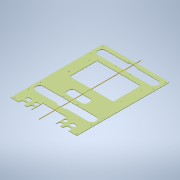
# Autodesk Inventor part: out_front
Saved by Autodesk Inventor 2020.2 (Build 242310000, 310)
## iProperties
Created: 2017-08-14
Part Number: out_front
Material: 一般
Document SubType Name: Modeling
Designer: gisen
Density: 1 g/cm^3
Appearance: クロム酸亜鉛 2
Author: gisen
Autodesk Inventor part; units mm, degrees
note: some values were not read from the file. Chosen so that the rebuilt part matches the saved one: offset side.
ref_plane "YZ Plane" through (0, 0, 0) normal (1, 0, 0) x (0, 1, 0)
ref_plane "XZ Plane" through (0, 0, 0) normal (0, 1, 0) x (-1, 0, 0)
ref_plane "XY Plane" through (0, 0, 0) normal (0, 0, 1) x (1, 0, 0)
sketch "スケッチ1" plane through (0, 0, 0) normal (0, 0, 1) x (1, 0, 0)
  line L0 (-165, 165) -> (165, 165)
  line L1 (165, 165) -> (165, -165)
  line L2 (165, -165) -> (-165, -165)
  line L3 (-165, -165) -> (-165, 165)
  line L4 (-165, 165) -> (165, -165) construction
  line L5 (165, 165) -> (-165, -165) construction
  circle A0 centre (-155, 155) radius 1.6
  circle A1 centre (-155, -155) radius 1.6
  circle A2 centre (155, -155) radius 1.6
  circle A3 centre (155, 155) radius 1.6
  point P0 (0, 0)
  dimension "d0" = 330
  dimension "d1" = 330
  dimension "d2" = 3.2
  dimension "d3" = 3.2
  dimension "d4" = 3.2
  dimension "d5" = 3.2
  dimension "d6" = 10
  dimension "d7" = 10
  dimension "d8" = 10
  dimension "d9" = 10
  constraints: 12 end point, 4 centre point, 4 point on line, 2 midpoint, 2 parallel, 1 horizontal, 1 perpendicular
  measures "d0" distance of L1.end L2.end
  measures "d1" distance of L0.end L1.end
  measures "d2" diameter of A0
  measures "d3" diameter of A1
  measures "d4" diameter of A2
  measures "d5" diameter of A3
  measures "d6" distance from line of A0.centre L0
  measures "d7" distance from line of L2 A1.centre
  measures "d8" distance from line of L2 A2.centre
  measures "d9" distance from line of L0 A3.centre
extrude "押し出し1" add sketch "スケッチ1" along normal blind 2
sketch "スケッチ2" plane through (0, 0, 2) normal (0, 0, 1) x (1, 0, 0)
  circle A0 centre (155, 155) radius 1.6 construction
  circle A1 centre (155, -155) radius 1.6 construction
  circle A2 centre (-155, -155) radius 1.6 construction
  circle A3 centre (-155, 155) radius 1.6 construction
  line L0 (165, 165) -> (-165, 165) construction
  line L1 (-165, 165) -> (-165, -165) construction
  line L2 (-165, -165) -> (165, -165) construction
  line L3 (165, -165) -> (165, 165) construction
  line L4 (165, 165) -> (-165, 165) construction
  line L5 (0, 165) -> (0, -165) construction
  line L6 (-108.5, 102) -> (108.5, 102)
  line L7 (108.5, 102) -> (108.5, -35)
  line L8 (108.5, -35) -> (-108.5, -35)
  line L9 (-108.5, -35) -> (-108.5, 102)
  line L10 (-108.5, 102) -> (108.5, -35) construction
  line L11 (108.5, 102) -> (-108.5, -35) construction
  line L12 (-125, -55) -> (125, -55)
  line L13 (125, -55) -> (125, -119.5)
  line L14 (125, -119.5) -> (-125, -119.5)
  line L15 (-125, -119.5) -> (-125, -55)
  line L16 (-125, -55) -> (125, -119.5) construction
  line L17 (125, -55) -> (-125, -119.5) construction
  point P0 (0, 0)
  point P1 (0, 33.5)
  point P2 (0, -87.25)
  dimension "d12" = 63
  dimension "d13" = 217
  dimension "d14" = 137
  dimension "d15" = 20
  dimension "d16" = 64.5
  dimension "d17" = 250
  constraints: 26 end point, 6 midpoint, 4 parallel, 2 horizontal, 2 perpendicular, 2 point on line
  measures "d12" distance between parallel lines of L6 L0
  measures "d13" distance of L6.start L6.end
  measures "d14" distance of L6.end L7.end
  measures "d15" distance between parallel lines of L12 L8
  measures "d16" distance of L12.end L13.end
  measures "d17" distance of L13.end L14.end
extrude "押し出し2" cut sketch "スケッチ2" against normal through all
sketch "スケッチ3" plane through (0, 0, 0) normal (0, 0, -1) x (-1, 0, 0)
  line L0 (108.5, 102) -> (108.5, -35) construction
  line L1 (-108.5, -35) -> (-108.5, 102) construction
  line L2 (108.5, -35) -> (108.5, 102) construction
  line L3 (108.5, -35) -> (-108.5, 102) construction
  line L4 (-108.5, -35) -> (108.5, 102) construction
  line L5 (122.5, 105.5) -> (-122.5, 105.5) construction
  line L6 (-122.5, 105.5) -> (-122.5, -38.5) construction
  line L7 (-122.5, -38.5) -> (122.5, -38.5) construction
  line L8 (122.5, -38.5) -> (122.5, 105.5) construction
  line L9 (122.5, 105.5) -> (-122.5, -38.5) construction
  line L10 (-122.5, 105.5) -> (122.5, -38.5) construction
  line L11 (165, 165) -> (-165, 165) construction
  circle A0 centre (129.75, -16.5) radius 2
  line L12 (0, -38.5) -> (0, 165) construction
  line L13 (-122.5, -38.5) -> (-122.5, 105.5) construction
  circle A1 centre (-129.75, -16.5) radius 2
  circle A2 centre (129.75, 83.5) radius 2
  circle A3 centre (-129.75, 83.5) radius 2
  circle A4 centre (129.75, 93) radius 1.5
  circle A5 centre (129.75, 74) radius 1.5
  circle A6 centre (129.75, -7) radius 1.5
  circle A7 centre (129.75, -26) radius 1.5
  circle A8 centre (-129.75, -26) radius 1.5
  circle A9 centre (-129.75, -7) radius 1.5
  circle A10 centre (-129.75, 74) radius 1.5
  circle A11 centre (-129.75, 93) radius 1.5
  point P0 (0, 0)
  point P1 (0, 33.5)
  dimension "d20" = 245
  dimension "d21" = 144
  dimension "d26" = 22
  dimension "d27" = 7.25
  dimension "d30" = 7.25
  dimension "d33" = 7.25
  dimension "d71" = 4
  dimension "d72" = 22
  dimension "d73" = 22
  dimension "d74" = 4
  dimension "d75" = 4
  dimension "d76" = 3
  dimension "d77" = 3
  dimension "d78" = 3
  dimension "d79" = 3
  dimension "d80" = 3
  dimension "d81" = 3
  dimension "d82" = 3
  dimension "d83" = 3
  dimension "d84" = 9.5
  dimension "d86" = 9.5
  dimension "d87" = 9.5
  dimension "d88" = 9.5
  dimension "d89" = 9.5
  dimension "d90" = 9.5
  dimension "d91" = 9.5
  dimension "d92" = 9.5
  constraints: 20 end point, 12 centre point, 8 vertical alignment, 5 midpoint, 2 parallel, 1 horizontal, 1 perpendicular, 1 symmetric about line
  measures "d20" distance of L7.end L6.end
  measures "d21" distance of L5.end L6.end
  measures "d26" distance from line of A0.centre L7
  measures "d27" distance from line of L8 A0.centre
  measures "d30" distance from line of L8 A2.centre
  measures "d33" distance from line of L6 A3.centre
  measures "d71" diameter of A1
  measures "d72" distance from line of L5 A2.centre
  measures "d73" distance from line of L5 A3.centre
  measures "d74" diameter of A3
  measures "d75" diameter of A2
  measures "d76" diameter of A4
  measures "d77" diameter of A5
  measures "d78" diameter of A6
  measures "d79" diameter of A7
  measures "d80" diameter of A8
  measures "d81" diameter of A9
  measures "d82" diameter of A10
  measures "d83" diameter of A11
  measures "d84" distance of A3.centre A11.centre
  measures "d86" distance of A3.centre A10.centre
  measures "d87" distance of A1.centre A9.centre
  measures "d88" distance of A1.centre A8.centre
  measures "d89" distance of A0.centre A7.centre
  measures "d90" distance of A0.centre A6.centre
  measures "d91" distance of A2.centre A4.centre
  measures "d92" distance of A2.centre A5.centre
extrude "押し出し3" cut sketch "スケッチ3" against normal through all contours A0 | A1 | A2 | A3
sketch "スケッチ4" plane through (0, 0, 2) normal (0, 0, 1) x (1, 0, 0)
  line L0 (165, -165) -> (165, 165) projected
  line L1 (-165, -165) -> (165, -165)
  line L2 (165, -165) -> (165, -272)
  line L3 (165, -272) -> (-165, -272)
  line L4 (-165, -272) -> (-165, -165)
  circle A0 centre (-155, 155) radius 1.6 projected
  circle A1 centre (155, 155) radius 1.6 projected
  circle A2 centre (-155, -155) radius 1.6 projected
  circle A3 centre (155, -155) radius 1.6 projected
  circle A4 centre (-155, -262) radius 2.5
  circle A5 centre (155, -262) radius 2.5
  circle A6 centre (-155, 178) radius 2.5
  circle A7 centre (155, 178) radius 2.5
  line L5 (-165, 188) -> (165, 188)
  line L6 (165, 188) -> (165, 165)
  line L7 (165, 165) -> (-165, 165)
  line L8 (-165, 165) -> (-165, 188)
  point P0 (0, 0)
  dimension "d35" = 107
  dimension "d40" = 10
  dimension "d41" = 10
  dimension "d42" = 5
  dimension "d43" = 5
  dimension "d44" = 5
  dimension "d45" = 5
  dimension "d46" = 10
  dimension "d47" = 10
  dimension "d48" = 23
  dimension "d49" = 10
  dimension "d50" = 10
  dimension "d51" = 10
  dimension "d52" = 10
  constraints: 16 end point, 4 centre point, 4 parallel, 2 horizontal, 2 perpendicular, 2 point on line, 1 coincident
  measures "d35" distance of L1.end L2.end
  measures "d40" distance from line of L3 A4.centre
  measures "d41" distance from line of L4 A4.centre
  measures "d42" diameter of A6
  measures "d43" diameter of A7
  measures "d44" diameter of A5
  measures "d45" diameter of A4
  measures "d46" distance from line of L3 A5.centre
  measures "d47" distance from line of L2 A5.centre
  measures "d48" distance of L7.end L5.start
  measures "d49" distance from line of A6.centre L5
  measures "d50" distance from line of L8 A6.centre
  measures "d51" distance from line of L5 A7.centre
  measures "d52" distance from line of L6 A7.centre
extrude "押し出し4" add sketch "スケッチ4" against normal up to surface (2 mm away)
sketch "スケッチ8" plane through (0, 0, 0) normal (0, 0, -1) x (-1, 0, 0)
  circle A0 centre (-72.25, -236.56) radius 7.94 projected
  circle A1 centre (-72.25, -262.06) radius 7.94 projected
  circle A2 centre (72.25, -236.24) radius 7.44 projected
  circle A3 centre (72.25, -261.74) radius 7.44 projected
  line L0 (29, -272) -> (29, -227) projected
  line L1 (29, -227) -> (-31, -227) projected
  line L2 (-31, -227) -> (-31, -272) projected
  ellipse E0 centre (-109.425, -236.08) end of major axis (-121.4458, -236.08) minor radius 8.5 projected
  ellipse E1 centre (-109.425, -262.32) end of major axis (-121.4458, -262.32) minor radius 8.5 projected
  ellipse E2 centre (109.425, -236.08) end of major axis (121.4458, -236.08) minor radius 8.5 projected
  ellipse E3 centre (109.425, -262.32) end of major axis (121.4458, -262.32) minor radius 8.5 projected
  point P0 (0, 0)
  constraints: 4 other
extrude "押し出し8" cut sketch "スケッチ8" against normal blind 10
sketch "スケッチ9" plane through (0, 0, 0) normal (0, 0, -1) x (-1, 0, 0)
  line L0 (-31, -227) -> (-31, -272) projected
  line L1 (29, -227) -> (-31, -227) projected
  line L2 (29, -272) -> (29, -227) projected
  line L3 (-31, -272) -> (29, -272)
  line L4 (165, -272) -> (-165, -272) projected
  point P0 (0, 0)
  constraints: 2 end point, 1 collinear
extrude "押し出し9" cut sketch "スケッチ9" against normal blind 10
sketch "スケッチ13" plane through (0, 0, 2) normal (0, 0, 1) x (1, 0, 0)
  line L0 (-130, -162.3) -> (130, -162.3) construction
  line L1 (-130, -142.3) -> (130, -142.3)
  line L2 (130, -182.3) -> (-130, -182.3)
  arc A0 (-130, -142.3) -> (-130, -182.3) centre (-130, -162.3) ccw
  arc A1 (130, -182.3) -> (130, -142.3) centre (130, -162.3) ccw
  line L3 (-165, -272) -> (-29, -272) projected
  point P0 (0, 0)
  point P1 (0, -162.3)
  dimension "d116" = 40
  dimension "d117" = 0
  dimension "d118" = 260
  dimension "d119" = 129.7
  constraints: 8 end point, 4 point on circle, 4 tangent, 2 centre point, 1 horizontal, 1 midpoint, 1 parallel
  measures "d116" diameter of A0
  measures "d117" horizontal distance of point (0, 0) point (0, -162.3)
  measures "d118" distance of L0.end L0.start
  measures "d119" distance between parallel lines of L1 L3
extrude "押し出し13" cut sketch "スケッチ13" against normal through all
sketch "スケッチ14" plane through (0, 0, 2) normal (0, 0, 1) x (1, 0, 0)
  line L0 (-130, 147.8) -> (130, 147.8) construction
  line L1 (-130, 167.8) -> (130, 167.8)
  line L2 (130, 127.8) -> (-130, 127.8)
  arc A0 (-130, 167.8) -> (-130, 127.8) centre (-130, 147.8) ccw
  arc A1 (130, 127.8) -> (130, 167.8) centre (130, 147.8) ccw
  arc A2 (-130, -142.3) -> (-130, -182.3) centre (-130, -162.3) ccw projected
  line L3 (-130, -142.3) -> (130, -142.3) projected
  line L4 (-130, 147.8) -> (-130, -162.3) construction
  line L5 (165, 188) -> (-165, 188) construction
  point P0 (0, 0)
  point P1 (0, 147.8)
  dimension "d125" = 60.2
  constraints: 10 end point, 4 point on circle, 4 tangent, 2 centre point, 2 parallel, 1 equal radius, 1 horizontal, 1 midpoint, 1 perpendicular
  measures "d125" distance between parallel lines of L2 L5
extrude "押し出し14" cut sketch "スケッチ14" against normal through all
sketch "スケッチ15" plane through (0, 0, 2) normal (0, 0, 1) x (1, 0, 0)
  line L0 (130, 127.8) -> (-130, 127.8) construction
  line L1 (-130, -142.3) -> (130, -142.3) construction
  line L2 (-35.5, 122.5) -> (35.5, 122.5) construction
  line L3 (35.5, 122.5) -> (35.5, 137.5) construction
  line L4 (35.5, 137.5) -> (-35.5, 137.5) construction
  line L5 (-35.5, 137.5) -> (-35.5, 122.5) construction
  line L6 (-35.5, 122.5) -> (35.5, 137.5) construction
  line L7 (35.5, 122.5) -> (-35.5, 137.5) construction
  line L8 (0, 130) -> (0, 127.8) construction
  line L9 (-35.5, -137) -> (35.5, -137) construction
  line L10 (35.5, -137) -> (35.5, -152) construction
  line L11 (35.5, -152) -> (-35.5, -152) construction
  line L12 (-35.5, -152) -> (-35.5, -137) construction
  line L13 (-35.5, -137) -> (35.5, -152) construction
  line L14 (35.5, -137) -> (-35.5, -152) construction
  line L15 (0, -144.5) -> (0, -142.3) construction
  circle A0 centre (-35.5, 137.5) radius 2.1
  circle A1 centre (-35.5, 122.5) radius 2.1
  circle A2 centre (35.5, 122.5) radius 2.1
  circle A3 centre (35.5, 137.5) radius 2.1
  circle A4 centre (-35.5, -137) radius 2.1
  circle A5 centre (-35.5, -152) radius 2.1
  circle A6 centre (35.5, -152) radius 2.1
  circle A7 centre (35.5, -137) radius 2.1
  point P0 (0, 0)
  dimension "d126" = 71
  dimension "d127" = 15
  dimension "d128" = 9.7
  dimension "d129" = 9.7
  dimension "d130" = 4.2
  constraints: 28 end point, 8 centre point, 8 coincident, 7 equal radius, 6 midpoint, 4 parallel, 4 perpendicular, 2 equal length, 2 horizontal
  measures "d126" distance of L4.end L3.end
  measures "d127" distance of L3.end L2.end
  measures "d128" distance between parallel lines of L4 L0
  measures "d129" distance between parallel lines of L1 L11
  measures "d130" diameter of A0
extrude "押し出し15" cut sketch "スケッチ15" against normal through all
sketch "スケッチ6" plane through (0, 0, 2) normal (0, 0, 1) x (1, 0, 0)
  circle A0 centre (-155, -262) radius 2.5 construction
  circle A1 centre (155, -262) radius 2.5 construction
  line L0 (-155, -262) -> (155, -262) construction
  line L1 (155, -262) -> (155, -132.3) construction
  line L2 (155, -132.3) -> (-155, -132.3) construction
  line L3 (-155, -132.3) -> (-155, -262) construction
  circle A2 centre (-155, -132.3) radius 2.5
  circle A3 centre (155, -132.3) radius 2.5
  arc A4 (130, -182.3) -> (130, -142.3) centre (130, -162.3) ccw projected
  line L4 (-130, -142.3) -> (130, -142.3) projected
  point P0 (0, 0)
  dimension "d61" = 129.7
  dimension "d155" = 10
  constraints: 8 end point, 3 coincident, 2 centre point, 2 equal radius, 2 parallel, 1 horizontal, 1 perpendicular
  measures "d61" distance of L0.end L1.end
  measures "d155" distance between parallel lines of L4 L2
extrude "押し出し6" cut sketch "スケッチ6" against normal through all
sketch "スケッチ16" plane through (0, 0, 2) normal (0, 0, 1) x (1, 0, 0)
  line L0 (130, 127.8) -> (-130, 127.8) construction
  line L1 (130, -182.3) -> (-130, -182.3) construction
  circle A0 centre (-155, 178) radius 2.5 construction
  circle A1 centre (-155, -132.3) radius 2.5 construction
  circle A2 centre (-155, -262) radius 2.5 construction
  circle A3 centre (155, -262) radius 2.5 construction
  circle A4 centre (155, -132.3) radius 2.5 construction
  circle A5 centre (155, 178) radius 2.5 construction
  line L2 (-155, 178) -> (-155, -262) construction
  line L3 (155, -262) -> (155, 178) construction
  circle A6 centre (-155, -192.3) radius 2.5
  circle A7 centre (155, -192.3) radius 2.5
  circle A8 centre (-155, 117.8) radius 2.5
  circle A9 centre (155, 117.8) radius 2.5
  point P0 (0, 0)
  dimension "d133" = 10
  dimension "d134" = 10
  dimension "d135" = 10
  dimension "d136" = 10
  constraints: 4 centre point, 4 end point, 4 equal radius, 4 point on line, 2 vertical
  measures "d133" distance from line of A8.centre L0
  measures "d134" distance from line of A9.centre L0
  measures "d135" distance from line of A6.centre L1
  measures "d136" distance from line of A7.centre L1
extrude "押し出し16" cut sketch "スケッチ16" against normal through all
sketch "スケッチ17" plane through (0, 0, 2) normal (0, 0, 1) x (1, 0, 0)
  line L0 (59.15, -254.725) -> (-59.15, -254.725)
  line L1 (-59.15, -254.725) -> (-59.15, -233.975)
  line L2 (-59.15, -233.975) -> (59.15, -233.975)
  line L3 (59.15, -233.975) -> (59.15, -254.725)
  line L4 (59.15, -254.725) -> (-59.15, -233.975) construction
  line L5 (-59.15, -254.725) -> (59.15, -233.975) construction
  line L6 (-165, -272) -> (-29, -272) projected
  line L7 (38.15, -216.7) -> (-38.15, -216.7)
  line L8 (-38.15, -216.7) -> (-38.15, -272)
  line L9 (-38.15, -272) -> (38.15, -272)
  line L10 (38.15, -272) -> (38.15, -216.7)
  line L11 (38.15, -216.7) -> (-38.15, -272) construction
  line L12 (-38.15, -216.7) -> (38.15, -272) construction
  point P0 (0, 0)
  point P1 (0, -244.35)
  dimension "d139" = 118.3
  dimension "d140" = 17.275
  dimension "d141" = 0
  dimension "d142" = 20.75
  dimension "d143" = 76.3
  constraints: 24 end point, 4 midpoint, 4 parallel, 2 horizontal, 2 perpendicular, 1 point on line
  measures "d139" distance of L0.start L0.end
  measures "d140" distance between parallel lines of L6 L0
  measures "d141" horizontal distance of point (0, 0) point (0, -244.35)
  measures "d142" distance of L0.end L1.end
  measures "d143" distance of L7.start L7.end
extrude "押し出し17" cut sketch "スケッチ17" against normal through all
sketch "スケッチ18" plane through (0, 0, 2) normal (0, 0, 1) x (1, 0, 0)
  line L0 (38.15, -233.975) -> (-38.15, -254.725) construction
  line L1 (-38.15, -254.725) -> (-38.15, -233.975) construction
  line L2 (38.15, -254.725) -> (38.15, -272) construction
  line L3 (-38.15, -233.975) -> (38.15, -254.725) construction
  line L4 (38.15, -216.7) -> (38.15, -233.975) construction
  line L5 (38.15, -254.725) -> (38.15, -233.975) construction
  line L6 (45.5, -266.6) -> (-45.5, -266.6) construction
  line L7 (-45.5, -266.6) -> (-45.5, -222.1) construction
  line L8 (-45.5, -222.1) -> (45.5, -222.1) construction
  line L9 (45.5, -222.1) -> (45.5, -266.6) construction
  line L10 (45.5, -266.6) -> (-45.5, -222.1) construction
  line L11 (-45.5, -266.6) -> (45.5, -222.1) construction
  circle A0 centre (-45.5, -266.6) radius 2.1
  circle A1 centre (-45.5, -222.1) radius 2.1
  circle A2 centre (45.5, -222.1) radius 2.1
  circle A3 centre (45.5, -266.6) radius 2.1
  point P0 (0, 0)
  point P1 (0, -244.35)
  dimension "d146" = 91
  dimension "d147" = 44.5
  dimension "d148" = 4.2
  dimension "d149" = 4.2
  dimension "d150" = 4.2
  dimension "d151" = 4.2
  constraints: 20 end point, 4 centre point, 4 coincident, 3 midpoint, 2 parallel, 1 collinear, 1 horizontal, 1 perpendicular, 1 vertical
  measures "d146" distance of L7.end L8.end
  measures "d147" distance of L6.end L7.end
  measures "d148" diameter of A0
  measures "d149" diameter of A1
  measures "d150" diameter of A2
  measures "d151" diameter of A3
extrude "押し出し18" cut sketch "スケッチ18" against normal through all
sketch "スケッチ20" plane through (0, 0, 2) normal (0, 0, 1) x (1, 0, 0)
  line L0 (-22.7689, 167.8) -> (-17.5, 172.8)
  line L1 (-17.5, 172.8) -> (17.5, 172.8)
  line L2 (17.5, 172.8) -> (22.7689, 167.8)
  line L3 (-130, 167.8) -> (130, 167.8) projected
  line L4 (-22.7689, 167.8) -> (22.7689, 167.8)
  point P0 (0, 0)
  point P1 (0, 172.8)
  dimension "d156" = 43.5
  dimension "d157" = 43.5
  dimension "d158" = 0
  dimension "d159" = 5
  dimension "d160" = 35
  constraints: 8 end point, 1 horizontal, 1 midpoint, 1 parallel, 1 point on line
  measures "d156" angle of L3 L0
  measures "d157" angle of L3 L2
  measures "d158" horizontal distance of point (0, 0) point (0, 172.8)
  measures "d159" distance between parallel lines of L3 L1
  measures "d160" distance of L0.end L1.end
extrude "押し出し19" cut sketch "スケッチ20" against normal through all
sketch "スケッチ21" plane through (0, 0, 2) normal (0, 0, 1) x (1, 0, 0)
  line L0 (130, 127.8) -> (-130, 127.8) construction
  line L1 (-130, -142.3) -> (130, -142.3) construction
  line L2 (0, 127.8) -> (0, -142.3) construction
  line L3 (0, -7.25) -> (-164.9219, -7.25) construction
  line L4 (-22.7689, 167.8) -> (-17.5, 172.8) construction
  line L5 (-17.5, 172.8) -> (17.5, 172.8) construction
  line L6 (17.5, 172.8) -> (22.7689, 167.8) construction
  line L7 (-22.7689, -182.3) -> (-17.5, -187.3)
  line L8 (-17.5, -187.3) -> (17.5, -187.3)
  line L9 (17.5, -187.3) -> (22.7689, -182.3)
  line L10 (-22.7689, -182.3) -> (22.7689, -182.3)
  line L11 (130, -182.3) -> (-130, -182.3) construction
  point P0 (0, 0)
  constraints: 12 end point, 4 symmetric about line, 3 midpoint, 1 collinear, 1 horizontal
extrude "押し出し20" cut sketch "スケッチ21" against normal through all
sketch "スケッチ22" plane through (0, 0, 2) normal (0, 0, 1) x (1, 0, 0)
  ellipse E0 centre (-109.425, -262.32) end of major axis (-97.4042, -262.32) minor radius 8.5 construction
  circle A0 centre (-72.25, -236.24) radius 7.44 construction
  circle A1 centre (-72.25, -261.74) radius 7.44 construction
  circle A2 centre (-72.25, -236.24) radius 8.94
  circle A3 centre (-72.25, -261.74) radius 9.44
  line L0 (-165, -272) -> (-38.15, -272) construction
  ellipse E1 centre (-111.5463, -262.32) end of major axis (-99.5255, -262.32) minor radius 8.5 construction
  line L1 (-111.5463, -262.32) -> (-109.425, -262.32) construction
  ellipse E2 centre (-109.425, -236.08) end of major axis (-97.4042, -236.08) minor radius 8.5 construction
  line L2 (-109.425, -236.08) -> (-109.425, -262.32) construction
  line L3 (-165, -272) -> (-165, 188) construction
  line L4 (-111.5463, -262.32) -> (-111.5463, -236.08) construction
  line L5 (-111.5463, -236.08) -> (-109.425, -236.08) construction
  ellipse E3 centre (-109.425, -236.08) end of major axis (-97.4042, -236.08) minor radius 8.5 construction
  ellipse E4 centre (-111.5463, -236.08) end of major axis (-99.5255, -236.08) minor radius 8.5 construction
  spline S0 degree 5 poles (-96.9042, -262.32) (-96.904, -261.2283) (-97.1336, -260.1332) (-97.5918, -259.1121) (-98.922, -257.1348) (-100.805, -255.6589) (-101.9079, -255.0151) (-104.3597, -253.934) (-106.9885, -253.4045) (-108.3892, -253.2672) (-111.1519, -253.268) (-113.8602, -253.8138) (-115.1582, -254.2165) (-117.4882, -255.2384) (-119.4794, -256.8104) (-120.3051, -257.6637) (-121.5772, -259.5523) (-122.0567, -261.7708) (-122.0567, -262.8692) (-121.5772, -265.0877) (-120.3051, -266.9763) (-119.4794, -267.8296) (-117.4882, -269.4016) (-115.1582, -270.4235) (-113.8602, -270.8262) (-111.1519, -271.372) (-108.3892, -271.3728) (-106.9885, -271.2355) (-104.3597, -270.706) (-101.9079, -269.6249) (-100.805, -268.9811) (-98.922, -267.5052) (-97.5918, -265.5279) (-97.1336, -264.5068) (-96.904, -263.4117) (-96.9042, -262.32) knots 0 0 0 0 0 0 0.080214 0.080214 0.080214 0.173201 0.173201 0.173201 0.275913 0.275913 0.275913 0.375087 0.375087 0.375087 0.460983 0.460983 0.460983 0.539017 0.539017 0.539017 0.624913 0.624913 0.624913 0.724087 0.724087 0.724087 0.826799 0.826799 0.826799 0.919786 0.919786 0.919786 1 1 1 1 1 1
  spline S1 degree 5 poles (-99.0255, -262.32) (-99.0253, -261.2283) (-99.2549, -260.1332) (-99.7132, -259.1121) (-101.0433, -257.1348) (-102.9263, -255.6589) (-104.0293, -255.0151) (-106.481, -253.934) (-109.1098, -253.4045) (-110.5105, -253.2672) (-113.2732, -253.268) (-115.9816, -253.8138) (-117.2795, -254.2165) (-119.6095, -255.2384) (-121.6007, -256.8104) (-122.4264, -257.6637) (-123.6985, -259.5523) (-124.178, -261.7708) (-124.178, -262.8692) (-123.6985, -265.0877) (-122.4264, -266.9763) (-121.6007, -267.8296) (-119.6095, -269.4016) (-117.2795, -270.4235) (-115.9816, -270.8262) (-113.2732, -271.372) (-110.5105, -271.3728) (-109.1098, -271.2355) (-106.481, -270.706) (-104.0293, -269.6249) (-102.9263, -268.9811) (-101.0433, -267.5052) (-99.7132, -265.5279) (-99.2549, -264.5068) (-99.0253, -263.4117) (-99.0255, -262.32) knots 0 0 0 0 0 0 0.080214 0.080214 0.080214 0.173201 0.173201 0.173201 0.275913 0.275913 0.275913 0.375087 0.375087 0.375087 0.460983 0.460983 0.460983 0.539017 0.539017 0.539017 0.624913 0.624913 0.624913 0.724087 0.724087 0.724087 0.826799 0.826799 0.826799 0.919786 0.919786 0.919786 1 1 1 1 1 1
  spline S2 degree 5 poles (-96.9042, -236.08) (-96.904, -234.9883) (-97.1336, -233.8932) (-97.5918, -232.8721) (-98.922, -230.8948) (-100.805, -229.4189) (-101.9079, -228.7751) (-104.3597, -227.694) (-106.9885, -227.1645) (-108.3892, -227.0272) (-111.1519, -227.028) (-113.8602, -227.5738) (-115.1582, -227.9765) (-117.4882, -228.9984) (-119.4794, -230.5704) (-120.3051, -231.4237) (-121.5772, -233.3123) (-122.0567, -235.5308) (-122.0567, -236.6292) (-121.5772, -238.8477) (-120.3051, -240.7363) (-119.4794, -241.5896) (-117.4882, -243.1616) (-115.1582, -244.1835) (-113.8602, -244.5862) (-111.1519, -245.132) (-108.3892, -245.1328) (-106.9885, -244.9955) (-104.3597, -244.466) (-101.9079, -243.3849) (-100.805, -242.7411) (-98.922, -241.2652) (-97.5918, -239.2879) (-97.1336, -238.2668) (-96.904, -237.1717) (-96.9042, -236.08) knots 0 0 0 0 0 0 0.080214 0.080214 0.080214 0.173201 0.173201 0.173201 0.275913 0.275913 0.275913 0.375087 0.375087 0.375087 0.460983 0.460983 0.460983 0.539017 0.539017 0.539017 0.624913 0.624913 0.624913 0.724087 0.724087 0.724087 0.826799 0.826799 0.826799 0.919786 0.919786 0.919786 1 1 1 1 1 1
  spline S3 degree 5 poles (-99.0255, -236.08) (-99.0253, -234.9883) (-99.2549, -233.8932) (-99.7132, -232.8721) (-101.0433, -230.8948) (-102.9263, -229.4189) (-104.0293, -228.7751) (-106.481, -227.694) (-109.1098, -227.1645) (-110.5105, -227.0272) (-113.2732, -227.028) (-115.9816, -227.5738) (-117.2795, -227.9765) (-119.6095, -228.9984) (-121.6007, -230.5704) (-122.4264, -231.4237) (-123.6985, -233.3123) (-124.178, -235.5308) (-124.178, -236.6292) (-123.6985, -238.8477) (-122.4264, -240.7363) (-121.6007, -241.5896) (-119.6095, -243.1616) (-117.2795, -244.1835) (-115.9816, -244.5862) (-113.2732, -245.132) (-110.5105, -245.1328) (-109.1098, -244.9955) (-106.481, -244.466) (-104.0293, -243.3849) (-102.9263, -242.7411) (-101.0433, -241.2652) (-99.7132, -239.2879) (-99.2549, -238.2668) (-99.0253, -237.1717) (-99.0255, -236.08) knots 0 0 0 0 0 0 0.080214 0.080214 0.080214 0.173201 0.173201 0.173201 0.275913 0.275913 0.275913 0.375087 0.375087 0.375087 0.460983 0.460983 0.460983 0.539017 0.539017 0.539017 0.624913 0.624913 0.624913 0.724087 0.724087 0.724087 0.826799 0.826799 0.826799 0.919786 0.919786 0.919786 1 1 1 1 1 1
  point P0 (0, 0)
  point P1 (72.25, -236.56)
  point P2 (72.25, -262.06)
  dimension "d170" = 0.5
  dimension "d173" = 0.5
  dimension "d175" = 0.5
  dimension "d176" = 0.5
  dimension "d165" = 1.5
  dimension "d166" = 2
  dimension "d174" = 2.1213
  constraints: 8 end point, 2 centre point, 2 coincident, 2 vertical, 1 horizontal, 1 perpendicular, 8 other
  measures "d165" radial gap between concentric circles of A0 A2
  measures "d166" radial gap between concentric circles of A1 A3
  measures "d174" distance of L1.start L1.end
extrude "押し出し21" cut sketch "スケッチ22" against normal up to surface (2 mm away)
sketch "スケッチ23" plane through (0, 0, 2) normal (0, 0, 1) x (1, 0, 0)
  circle A0 centre (-72.25, -261.74) radius 9.44 construction
  line L0 (-72.25, -261.74) -> (-165, -261.74) construction
  line L1 (-165, 188) -> (-165, -272) construction
  line L2 (-165, -272) -> (-38.15, -272) projected
  line L3 (-81.69, -261.74) -> (-62.81, -261.74)
  line L4 (-62.81, -261.74) -> (-62.81, -272)
  line L5 (-62.81, -272) -> (-81.69, -272)
  line L6 (-81.69, -272) -> (-81.69, -261.74)
  line L7 (-124.0413, -261.74) -> (-96.93, -261.74)
  line L8 (-96.93, -261.74) -> (-96.93, -272)
  line L9 (-96.93, -272) -> (-124.0413, -272)
  line L10 (-124.0413, -272) -> (-124.0413, -261.74)
  circle A1 centre (-72.25, -261.74) radius 9.44 projected
  point P0 (0, 0)
  constraints: 18 end point, 5 point on line, 4 parallel, 3 horizontal, 2 perpendicular, 2 point on circle, 1 horizontal alignment, 5 other
extrude "押し出し22" cut sketch "スケッチ23" against normal through all contours L10 L7 L8 L2 | L6 A1 L4 L2 | L3 A1 picked at (-70.0316, -267.8786)
ref_plane "作業平面1" through (0, -272, 0) normal (-1, 0, 0) x (0, 0, 1)
mirror "ミラー1" about plane through (0, -272, 0) normal (-1, 0, 0) of "押し出し21", "押し出し22"
sketch "スケッチ24" plane through (0, 0, 2) normal (0, 0, 1) x (1, 0, 0)
  line L0 (-164.6, 187.6) -> (164.6, 187.6)
  line L1 (164.6, 187.6) -> (164.6, -271.6)
  line L2 (164.6, -271.6) -> (-164.6, -271.6)
  line L3 (-164.6, -271.6) -> (-164.6, 187.6)
  line L4 (124.0413, -272) -> (165, -272) projected
  line L5 (165, -272) -> (165, 188) projected
  line L6 (-165, 188) -> (-165, -272) projected
  line L7 (165, 188) -> (-165, 188) projected
  point P0 (0, 0)
  dimension "d181" = 0.4
  dimension "d182" = 0.4
  dimension "d183" = 0.4
  dimension "d184" = 0.4
  constraints: 8 end point, 2 parallel, 1 horizontal, 1 perpendicular
  measures "d181" distance between parallel lines of L4 L2
  measures "d182" distance between parallel lines of L5 L1
  measures "d183" distance between parallel lines of L6 L3
  measures "d184" distance between parallel lines of L7 L0
extrude "押し出し23" cut sketch "スケッチ24" against normal through all keep common part
sketch "スケッチ26" plane through (0, 0, 2) normal (0, 0, 1) x (1, 0, 0)
  line L0 (-38.15, -271.6) -> (-62.81, -271.6) projected
  line L1 (-59.15, -271.6) -> (-59.15, -216.7)
  line L2 (-59.15, -233.975) -> (-59.15, -254.725) projected
  line L3 (-59.15, -216.7) -> (59.15, -216.7)
  line L4 (59.15, -216.7) -> (59.15, -271.6)
  line L5 (59.15, -271.6) -> (-59.15, -271.6)
  line L6 (-59.15, -254.725) -> (-59.15, -233.975) projected
  line L7 (-38.15, -216.7) -> (38.15, -216.7) projected
  line L8 (59.15, -233.975) -> (59.15, -254.725) projected
  point P0 (0, 0)
  constraints: 8 end point, 4 collinear, 2 perpendicular, 1 horizontal, 1 point on line
extrude "押し出し25" cut sketch "スケッチ26" against normal blind 2
sketch "スケッチ27" plane through (0, 0, 0) normal (0, 0, -1) x (-1, 0, 0)
  arc A0 (-38.35, -79.7) -> (-51.6, -92.95) centre (-38.35, -92.95) ccw
  line L0 (-38.35, -79.7) -> (38.35, -79.7)
  arc A1 (51.6, -92.95) -> (38.35, -79.7) centre (38.35, -92.95) ccw
  line L1 (51.6, -92.95) -> (51.6, -106.25)
  arc A2 (38.35, -119.5) -> (51.6, -106.25) centre (38.35, -106.25) ccw
  line L2 (125, -119.5) -> (-125, -119.5)
  arc A3 (-51.6, -106.25) -> (-38.35, -119.5) centre (-38.35, -106.25) ccw
  line L3 (-51.6, -106.25) -> (-51.6, -92.95)
  line L4 (-125, -55) -> (125, -55)
  line L5 (-125, -119.5) -> (-125, -55)
  line L6 (125, -55) -> (125, -119.5)
  point P0 (0, 0)
  point P1 (38.35, -79.7)
extrude "押し出し26" add sketch "スケッチ27" against normal blind 2 contours A0 L3 A3 L2 L5 L4 L6 A2 L1 A1 L0
